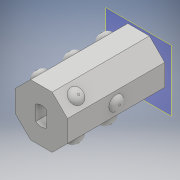
# Autodesk Inventor part: 8-Lados
Saved by Autodesk Inventor 2017 SP1 (Build 210196100, 196)
## iProperties
Created: 2017-08-27
Part Number: 8-Lados
Material: Generic
Document SubType Name: Modeling
Designer: Emanuel Suriano
Density: 1 g/cm^3
Appearance: Default
Author: Emanuel Suriano
## iProperties of the stored document 8-Lados_3DPrint.ipt
Created: 2017-08-27
Part Number: 8-Lados_3DPrint
Material: Generic
Document SubType Name: Modeling
Designer: Emanuel Suriano
Density: 1 g/cm^3
Appearance: Default
Author: Emanuel Suriano
Autodesk Inventor part; units mm, degrees
ref_plane "YZ Plane" through (0, 0, 0) normal (1, 0, 0) x (0, 1, 0)
ref_plane "XZ Plane" through (0, 0, 0) normal (0, 1, 0) x (-1, 0, 0)
ref_plane "XY Plane" through (0, 0, 0) normal (0, 0, 1) x (1, 0, 0)
sketch "Sketch3" plane through (0, 0, 0) normal (0, 1, 0) x (-1, 0, 0)
  line L0 (-3, -7.2426) -> (-7.2426, -3)
  line L1 (-7.2426, -3) -> (-7.2426, 3)
  line L2 (-7.2426, 3) -> (-3, 7.2426)
  line L3 (-3, 7.2426) -> (3, 7.2426)
  line L4 (3, 7.2426) -> (7.2426, 3)
  line L5 (7.2426, 3) -> (7.2426, -3)
  line L6 (7.2426, -3) -> (3, -7.2426)
  line L7 (3, -7.2426) -> (-3, -7.2426)
  point P0 (0, 0)
  point P1 (0, 0)
  dimension "d3" = 6
  constraints: 16 end point, 1 coincident, 17 other
  measures "d3" distance of L6.end L0.start
extrude "Extrusion2" add sketch "Sketch3" along normal blind 27
sketch "Sketch4" plane through (7.2426, 0, 3) normal (0.7071068, 0, 0.7071068) x (0.7071068, 0, -0.7071068)
  circle A0 centre (-3, 4.5) radius 2
  point P0 (-3, 0)
  dimension "d6" = 4
  dimension "d7" = 4.5
  constraints: 1 centre point
  measures "d6" diameter of A0
  measures "d7" distance of point (-3, 0) A0.centre
sketch "Sketch5" plane through (7.2426, 0, 3) normal (1, 0, 0) x (0, 0, -1)
  circle A0 centre (3, 13.5) radius 2
  point P0 (3, 0)
  dimension "d8" = 4
  dimension "d9" = 13.5
  constraints: 1 centre point
  measures "d8" diameter of A0
  measures "d9" distance of point (3, 0) A0.centre
sketch "Sketch6" plane through (3, 0, -7.2426) normal (0.7071068, 0, -0.7071068) x (-0.7071068, 0, -0.7071068)
  circle A0 centre (-3, 4.5) radius 2
  circle A1 centre (-3, 13.5) radius 2
  point P0 (-3, 0)
  dimension "d10" = 4
  dimension "d11" = 4
  dimension "d12" = 4.5
  dimension "d13" = 9
  constraints: 2 centre point
  measures "d10" diameter of A0
  measures "d11" diameter of A1
  measures "d12" distance of point (-3, 0) A0.centre
  measures "d13" distance of A0.centre A1.centre
sketch "Sketch7" plane through (3, 0, -7.2426) normal (0, 0, -1) x (-1, 0, 0)
  circle A0 centre (3, 22.5) radius 2
  point P0 (3, 0)
  dimension "d14" = 4
  dimension "d15" = 22.5
  constraints: 1 centre point
  measures "d14" diameter of A0
  measures "d15" distance of point (3, 0) A0.centre
sketch "Sketch8" plane through (-7.2426, 0, -3) normal (-0.7071068, 0, -0.7071068) x (-0.7071068, 0, 0.7071068)
  circle A0 centre (-3, 4.5) radius 2
  circle A1 centre (-3, 22.5) radius 2
  point P0 (-3, 0)
  dimension "d16" = 4
  dimension "d17" = 4.5
  dimension "d18" = 4
  dimension "d19" = 22.5
  constraints: 2 centre point
  measures "d16" diameter of A0
  measures "d17" distance of point (-3, 0) A0.centre
  measures "d18" diameter of A1
  measures "d19" distance of point (-3, 0) A1.centre
sketch "Sketch9" plane through (-7.2426, 0, -3) normal (-1, 0, 0) x (0, 0, 1)
  circle A0 centre (3, 13.5) radius 2
  circle A1 centre (3, 22.5) radius 2
  point P0 (3, 0)
  dimension "d20" = 4
  dimension "d21" = 4
  dimension "d22" = 13.5
  dimension "d23" = 22.5
  constraints: 2 centre point
  measures "d20" diameter of A0
  measures "d21" diameter of A1
  measures "d22" distance of point (3, 0) A0.centre
  measures "d23" distance of A1.centre point (3, 0)
sketch "Sketch10" plane through (-3, 0, 7.2426) normal (-0.7071068, 0, 0.7071068) x (0.7071068, 0, 0.7071068)
  circle A0 centre (-3, 4.5) radius 2
  circle A1 centre (-3, 13.5) radius 2
  circle A2 centre (-3, 22.5) radius 2
  point P0 (-3, 0)
  dimension "d24" = 4
  dimension "d25" = 4
  dimension "d26" = 4
  dimension "d27" = 4.5
  dimension "d28" = 9
  dimension "d29" = 9
  constraints: 3 centre point
  measures "d24" diameter of A0
  measures "d25" diameter of A1
  measures "d26" diameter of A2
  measures "d27" distance of point (-3, 0) A0.centre
  measures "d28" distance of A0.centre A1.centre
  measures "d29" distance of A1.centre A2.centre
extrude "Extrusion3" add sketch "Sketch4" along normal blind 1
extrude "Extrusion4" add sketch "Sketch5" along normal blind 1
extrude "Extrusion5" add sketch "Sketch6" along normal blind 1
extrude "Extrusion6" add sketch "Sketch7" along normal blind 1
extrude "Extrusion7" add sketch "Sketch8" along normal blind 1
extrude "Extrusion8" add sketch "Sketch9" along normal blind 1
extrude "Extrusion9" add sketch "Sketch10" along normal blind 1
fillet "Fillet1" radius 2 12 edges at (-7.2426, 22.5, 4.4142) (-7.2426, 13.5, 4.4142) (-7.2426, 4.5, 4.4142) (-8.2426, 13.5, -2) (-8.2426, 22.5, -2) (-4.4142, 22.5, -7.2426) (-4.4142, 4.5, -7.2426) (2, 22.5, -8.2426) (7.2426, 13.5, -4.4142) (7.2426, 4.5, -4.4142) (8.2426, 13.5, 2) (4.4142, 4.5, 7.2426)
ref_plane "Work Plane1" through (7.2426, 27, -3) normal (0, 1, 0) x (0, 0, -1)
sketch "Sketch12" plane through (7.2426, 27, -3) normal (0, 1, 0) x (0, 0, -1)
  point P0 (-3, 7.2426)
sketch "Sketch13" plane through (7.2426, 27, -3) normal (0, 1, 0) x (0, 0, -1)
  circle A0 centre (-3, 7.2426) radius 2.6
  line L0 (-5.0875, 5.6926) -> (-0.9125, 5.6926)
  line L1 (-5.0875, 8.7926) -> (-0.9125, 8.7926)
  dimension "d52" = 5.2
  dimension "d53" = 1.55
  dimension "d54" = 1.55
  constraints: 4 end point, 4 point on circle, 1 centre point, 1 coincident, 1 horizontal, 1 parallel
  measures "d52" diameter of A0
  measures "d53" distance from line of point (-3, 7.243) L0
  measures "d54" distance from line of point (-3, 7.243) L1
extrude "Extrusion10" cut sketch "Sketch13" against normal blind 58.75 contours A0 L0 L1
body "Solid2"
